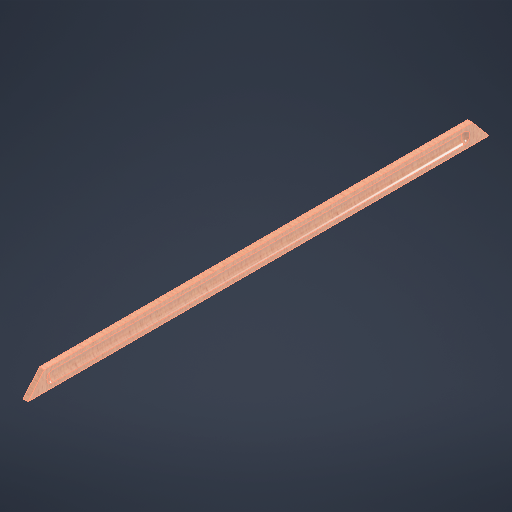
# Autodesk Inventor part: BASE_SIDEK_TREBUCHET
Saved by Autodesk Inventor 2026.2 (Build 302298010, 298A)
## iProperties
Created: 2026-02-18
Part Number: BASE_SIDEK_TREBUCHET
Material: Wood (Oak)
Document SubType Name: Modeling
Designer: 4aida
Density: 0.76 g/cm^3
Appearance: White Oak - Natural Medium Gloss
Mass: 176.907 g
Surface Area: 869.907 cm^2
Volume: 232.772 cm^3
Author: 4aida
Autodesk Inventor part; units mm, degrees
ref_plane "YZ Plane" through (0, 0, 0) normal (1, 0, 0) x (0, 1, 0)
ref_plane "XZ Plane" through (0, 0, 0) normal (0, 1, 0) x (-1, 0, 0)
ref_plane "XY Plane" through (0, 0, 0) normal (0, 0, 1) x (1, 0, 0)
sketch "Sketch1" plane through (0, 0, 0) normal (1, 0, 0) x (0, 1, 0)
  line L0 (-19.05, -447.675) -> (19.05, -447.675) construction
  line L1 (19.05, -447.675) -> (19.05, 447.675)
  line L2 (19.05, 447.675) -> (-19.05, 447.675) construction
  line L3 (-19.05, 447.675) -> (-19.05, -447.675)
  line L4 (-19.05, -447.675) -> (19.05, 447.675) construction
  line L5 (19.05, -447.675) -> (-19.05, 447.675) construction
  line L6 (-19.05, 447.675) -> (19.05, 415.7053)
  line L7 (-19.05, -447.675) -> (19.05, -415.7053)
  point P0 (0, 0)
  dimension "d0" = 895.35
  dimension "d1" = 38.1
  dimension "d16" = 40
  dimension "d17" = 40
  constraints: 16 end point, 2 midpoint, 2 parallel, 2 point on line, 1 horizontal, 1 perpendicular
  measures "d0" distance of L0.end L1.end
  measures "d1" distance of L1.end L2.end
  measures "d16" angle of L2 L6
  measures "d17" angle of L7 L0
extrude "Extrusion1" add sketch "Sketch1" along normal blind 9.525
sketch "Sketch3" plane through (0, 0, 0) normal (0, 0, 1) x (1, 0, 0)
  circle A0 centre (15.875, 0) radius 12.7
  point P0 (0, 0)
  point P1 (9.525, -19.05)
  dimension "d11" = 25.4
  dimension "d12" = 6.35
  constraints: 1 centre point, 1 horizontal alignment
  measures "d11" diameter of A0
  measures "d12" horizontal distance of A0.centre point (9.525, -19.05)
extrude "Extrusion3" cut sketch "Sketch3" along normal mid plane 825
fillet "Fillet1" radius 12.7 2 edges at (3.175, 0, -412.5) (3.175, 0, 412.5)
body "Solid1"
